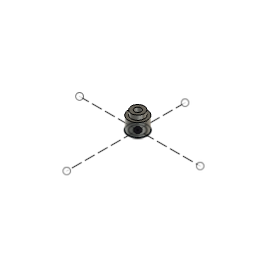
sphere2_disk_front v3 (Autodesk Fusion 360 design; units mm, degrees)
Autodesk Fusion 360 part; units mm, degrees
sketch "Skizze1" plane through (0, 0, 0) normal (0, 0, 1) x (1, 0, 0)
  line L0 (-31.5508, 0) -> (33.8224, 0) construction
  line L1 (0, 25.6192) -> (0, -38.4919) construction
  circle A0 centre (0, 0) radius 1.75
  circle A1 centre (0, 0) radius 3.5
  circle A2 centre (0, 0) radius 5
  dimension "d1" = 3.5
  dimension "d2" = 7
  dimension "d3" = 10
  constraint horizontal L0
  constraint coincident A0.centre L0
  constraint vertical L1
  constraint coincident A0.centre L1
  constraint coincident A0.centre A1.centre
  measures "d1" diameter of A0
  measures "d2" diameter of A1
  measures "d3" diameter of A2
extrude "Extrusion1" add sketch "Skizze1" along normal blind 7 contours A1 | A2
extrude "Extrusion2" add sketch "Skizze1" along normal blind 9.5 contours A1
extrude "Extrusion3" cut sketch "Skizze1" along normal blind 3 contours A1
